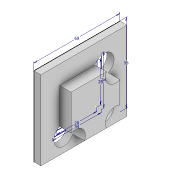
# Autodesk Inventor part: Cube_Insert_Motion_adapter_srew
Saved by Autodesk Inventor 2022 (Build 260153000, 153)
## iProperties
Created: 2023-06-30
Part Number: Cube_Insert_Motion_adapter_srew
Material: Generisch
Document SubType Name: Modeling
Designer: UC2
Density: 1 g/cm^3
Appearance: Vorgabe
Author: UC2
Autodesk Inventor part; units mm, degrees
ref_plane "YZ Plane" through (0, 0, 0) normal (1, 0, 0) x (0, 1, 0)
ref_plane "XZ Plane" through (0, 0, 0) normal (0, 1, 0) x (-1, 0, 0)
ref_plane "XY Plane" through (0, 0, 0) normal (0, 0, 1) x (1, 0, 0)
sketch "Skizze1" plane through (0, 0, 0) normal (1, 0, 0) x (0, 1, 0)
  line L0 (14, 14) -> (-14, 14)
  line L1 (-14, 14) -> (-14, -14)
  line L2 (-14, -14) -> (14, -14)
  line L3 (14, -14) -> (14, 14)
  line L4 (14, 14) -> (-14, -14) construction
  line L5 (-14, 14) -> (14, -14) construction
  line L6 (17, 17) -> (-17, 17)
  line L7 (-17, 17) -> (-17, -17)
  line L8 (-17, -17) -> (17, -17)
  line L9 (17, -17) -> (17, 17)
  line L10 (17, 17) -> (-17, -17) construction
  line L11 (-17, 17) -> (17, -17) construction
  line L12 (-25, 30) -> (30, 30)
  line L13 (30, 30) -> (30, -30)
  line L14 (30, -30) -> (-25, -30)
  line L15 (-25, -30) -> (-25, 30)
  point P0 (0, 0)
  dimension "d0" = 28
  dimension "d1" = 28
  dimension "d2" = 34
  dimension "d3" = 34
  dimension "d4" = 55
  dimension "d5" = 60
  constraints: 32 end point, 6 parallel, 4 midpoint, 3 horizontal, 3 perpendicular
  measures "d0" distance of L2.end L1.end
  measures "d1" distance of L1.end L0.end
  measures "d2" distance of L8.end L7.end
  measures "d3" distance of L7.end L6.end
  measures "d4" distance of L13.end L14.end
  measures "d5" distance of L12.end L13.end
extrude "Extrusion1" add sketch "Skizze1" along normal blind 13 contours L3 L2 L1 L0 | L9 L8 L7 L6
sketch "Skizze2" plane through (13, 0, 0) normal (1, 0, 0) x (0, 0, -1)
  point P0 (0, 0)
extrude "Extrusion2" add sketch "Skizze1" along normal blind 5 contours L12 L13 L14 L15
hole "Bohrung1" at (0, 14, -14) at (0, -14, 14) at (0, -14, -14) direction (1, 0, 0) diameter 14 end through all
